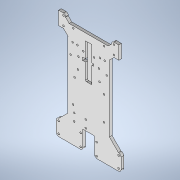
# Autodesk Inventor part: Основа робота
Saved by Autodesk Inventor 2020 (Build 240168000, 168)
## iProperties
Created: 2021-02-28
Part Number: Основа робота
Material: Типовые
Document SubType Name: Обычные детали
Designer: Антон
Density: 1 g/cm^3
Appearance: По умолчанию
Mass: 52.0111 g
Surface Area: 352.197 cm^2
Volume: 52.0111 cm^3
Sheet Metal Rule: По умолчанию
Author: Антон
Autodesk Inventor part; units mm, degrees
ref_plane "YZ Plane" through (0, 0, 0) normal (1, 0, 0) x (0, 1, 0)
ref_plane "XZ Plane" through (0, 0, 0) normal (0, 1, 0) x (-1, 0, 0)
ref_plane "XY Plane" through (0, 0, 0) normal (0, 0, 1) x (1, 0, 0)
sketch "Эскиз1" plane through (0, 0, 0) normal (0, 0, 1) x (1, 0, 0)
  line L0 (0, 0) -> (39, 0)
  line L1 (39, 0) -> (39, 194.6)
  line L2 (39, 194.6) -> (0, 194.6)
  line L3 (0, 194.6) -> (0, 0)
  line L4 (0, 0) -> (-22.05, 0)
  line L5 (-22.05, 0) -> (-22.05, 30.3)
  line L6 (-22.05, 30.3) -> (0, 30.3)
  line L7 (0, 30.3) -> (0, 0)
  line L8 (-22.05, 0) -> (-17.5, 0)
  line L9 (-17.5, 0) -> (-17.5, 4.55)
  line L10 (-17.5, 4.55) -> (-17.5, 25.75)
  circle A0 centre (-17.5, 25.75) radius 1.6
  circle A1 centre (-17.5, 4.55) radius 1.6
  line L11 (39, 0) -> (28, 0)
  line L12 (28, 0) -> (28, 35)
  line L13 (28, 35) -> (39, 35)
  line L14 (39, 35) -> (39, 0)
  line L15 (28, 4) -> (24, 4)
  line L16 (28, 26.9) -> (24, 26.9)
  circle A2 centre (24, 26.9) radius 1.6
  circle A3 centre (24, 4) radius 1.6
  line L17 (39, 154.3) -> (-0.05, 154.3)
  line L18 (-0.05, 154.3) -> (-0.05, 122.8)
  line L19 (-0.05, 122.8) -> (39, 122.8)
  line L20 (39, 122.8) -> (39, 154.3)
  line L21 (-0.05, 154.3) -> (4.95, 154.3)
  line L22 (4.95, 154.3) -> (4.95, 136.3)
  line L23 (4.95, 136.3) -> (-0.05, 136.3)
  line L24 (-0.05, 136.3) -> (-0.05, 154.3)
  line L25 (39, 122.8) -> (18.5177, 122.8)
  line L26 (18.5177, 122.8) -> (18.5177, 132.8)
  line L27 (18.5177, 132.8) -> (39, 132.8)
  line L28 (39, 132.8) -> (39, 122.8)
  line L29 (18.5177, 132.8) -> (9.8575, 127.8)
  line L30 (9.8575, 127.8) -> (4.95, 136.3)
  line L31 (4.95, 136.3) -> (13.6103, 141.3)
  line L32 (13.6103, 141.3) -> (18.5177, 132.8)
  line L33 (18.5177, 122.8) -> (9.8575, 127.8)
  line L34 (13.6103, 141.3) -> (4.95, 154.3)
  line L35 (39, 194.6) -> (39, 154.3)
  circle A4 centre (4.95, 145.3) radius 1.6
  line L36 (18.5177, 132.8) -> (28.7497, 132.8)
  line L37 (28.7497, 132.8) -> (28.7497, 162.65)
  circle A5 centre (28.7497, 162.65) radius 1.6
  line L38 (19.75, 167.25) -> (19.75, 149.25)
  circle A6 centre (19.75, 149.25) radius 1.6
  line L39 (0, 167.25) -> (19.75, 167.25)
  line L40 (19.75, 167.25) -> (17.75, 167.25)
  circle A7 centre (17.75, 167.25) radius 1.6
  line L41 (17.75, 167.25) -> (8.75, 167.25)
  circle A8 centre (8.75, 167.25) radius 1.6
  line L42 (34.9997, 132.8) -> (34.9997, 135.85)
  circle A9 centre (34.9997, 135.85) radius 2.5
  line L43 (39, 137.8498) -> (36.5, 137.8498)
  line L44 (36.5, 137.8498) -> (36.5, 133.8502)
  line L45 (36.5, 133.8502) -> (39, 133.8502)
  line L46 (39, 133.8502) -> (39, 137.8498)
  line L47 (39, 194.6) -> (39, 190.6)
  line L48 (39, 190.6) -> (10, 190.6)
  circle A10 centre (10, 190.6) radius 1.6
  line L49 (39, 194.6) -> (34, 194.6)
  line L50 (34, 194.6) -> (18, 194.6)
  line L51 (0, 181.3) -> (-17.75, 181.3)
  line L52 (-17.75, 181.3) -> (-17.75, 206.3)
  line L53 (-17.75, 206.3) -> (0, 206.3)
  line L54 (0, 206.3) -> (0, 181.3)
  line L55 (-17.75, 193.8) -> (-8.55, 193.8)
  line L56 (-8.55, 202.3) -> (-8.55, 185.3)
  circle A11 centre (-8.55, 202.3) radius 1.6
  circle A12 centre (-8.55, 185.3) radius 1.6
  line L57 (0, 206.3) -> (-4.55, 206.3)
  line L58 (-4.55, 206.3) -> (-4.55, 194.6)
  line L59 (-4.55, 194.6) -> (0, 194.6)
  line L60 (0, 194.6) -> (0, 206.3)
  line L61 (-8.55, 193.8) -> (-8.05, 193.8)
  circle A13 centre (18.5177, 127.8) radius 1.6
  point P0 (0, 30.3)
  point P1 (28, 0)
  point P2 (39, 35)
  point P3 (36.5, 135.85)
  point P4 (36.5, 133.8502)
  point P5 (37.1648, 143.2)
  point P6 (37.75, 137.8498)
  point P7 (36.5, 143.9498)
  point P8 (36.5, 133.8502)
  point P9 (0, 182.1)
  point P10 (0, 181.3)
  point P11 (0, 194.6)
  point P12 (0, 194.6)
  point P13 (-4.55, 206.3)
  dimension "d293" = 5
  dimension "d0" = 39
  dimension "d1" = 194.6
  dimension "d191" = 22.05
  dimension "d192" = 30.3
  dimension "d207" = 4.55
  dimension "d208" = 4.55
  dimension "d209" = 21.2
  dimension "d210" = 11
  dimension "d211" = 35
  dimension "d215" = 4
  dimension "d270" = 39.05
  dimension "d271" = 31.5
  dimension "d273" = 18
  dimension "d274" = 5
  dimension "d276" = 10
  dimension "d277" = 60
  dimension "d278" = 10
  dimension "d280" = 40.3
  dimension "d283" = 10.232
  dimension "d284" = 29.85
  dimension "d285" = 18
  dimension "d286" = 19.75
  dimension "d287" = 27.35
  dimension "d288" = 2
  dimension "d289" = 9
  dimension "d290" = 3.2
  dimension "d292" = 16.482
  dimension "d294" = 3.05
  dimension "d305" = 2.5
  dimension "d309" = 29
  dimension "d310" = 3.2
  dimension "d311" = 3.2
  dimension "d316" = 17.75
  dimension "d317" = 25
  dimension "d320" = 9.2
  dimension "d321" = 3.2
  dimension "d322" = 17
  dimension "d324" = 13.3
  dimension "d325" = 4
  dimension "d333" = 4.55
  dimension "d342" = 0.5
  dimension "d387" = 22.9
  dimension "d388" = 4
  dimension "d404" = 3.2
  constraints: 124 end point, 21 parallel, 15 perpendicular, 14 horizontal, 13 centre point, 13 point on line, 12 coincident, 8 equal radius, 6 midpoint, 3 collinear, 2 vertical, 1 horizontal alignment, 3 other
  measures "d0" distance of L2.end L1.end
  measures "d1" distance of L1.end L0.end
  measures "d191" distance of L5.end L6.end
  measures "d192" distance of L4.end L5.end
  measures "d207" distance of L4.end L8.end
  measures "d208" distance of L8.end L9.end
  measures "d209" distance of L9.end L10.end
  measures "d210" distance of L12.end L13.end
  measures "d211" distance of L11.end L12.end
  measures "d215" distance of L16.start L16.end
  measures "d270" distance of L19.end L18.end
  measures "d271" distance of L18.end L17.end
  measures "d273" distance of L21.end L22.end
  measures "d274" distance between parallel lines of L18 L22
  measures "d276" distance between parallel lines of L25 L27
  measures "d277" angle of L22 L31
  measures "d278" distance between parallel lines of L30 L32
  measures "d280" distance of L1.end L17.start
  measures "d283" distance of L26.end L36.end
  measures "d284" distance of L36.end L37.end
  measures "d285" distance of L38.start L38.end
  measures "d286" distance of L39.start L38.start
  measures "d287" distance between parallel lines of L2 L39
  measures "d288" distance of L38.start L40.end
  measures "d289" distance of L41.start L41.end
  measures "d290" diameter of A2
  measures "d292" distance between parallel lines of L26 L42
  measures "d294" distance of L42.start L42.end
  measures "d305" distance of L45.end L44.end
  measures "d309" distance of L47.end L48.end
  measures "d310" diameter of A8
  measures "d311" diameter of A10
  measures "d316" distance of L52.end L53.end
  measures "d317" distance of L51.end L52.end
  measures "d320" distance of L55.end L55.start
  measures "d321" diameter of A11
  measures "d322" distance of L56.end L56.start
  measures "d324" distance between parallel lines of L2 L51
  measures "d325" distance from line of L49.end L48
  measures "d333" distance of L59.end L58.end
  measures "d342" distance of L61.end L55.end
  measures "d387" distance of A3.centre A2.centre
  measures "d388" distance between parallel lines of L0 L15
  measures "d404" diameter of A4
extrude "Выдавливание1" add sketch "Эскиз1" along normal blind 5 contours L3 L19 L1 L13 L12 L0 | L4 L5 L6 L3 | L3 L23 L30 L33 L19 | L3 L17 L22 A4 L23 | L26 A13 L27 L1 L19 | L33 L29 L26 A13 | L3 L39 A8 A7 L38 L17 | L31 L32 L29 L30 | L22 A4 L34 L31 | L27 L42 A9 L45 L1 | L3 L2 L1 L17 L38 L39 A7 A8 | L17 L37 L27 L32 L34 | L45 A9 L43 L1 | L27 L37 L17 L1 L43 A9 L42 | L51 L52 L53 L58 L59 L3 | L44 A9 | A9 L44
mirror "Зеркальное отражение1" about plane through (39, 35, 0) normal (1, 0, 0) of "Выдавливание1"
sketch "Эскиз18" plane through (0, 0, 5) normal (0, 0, 1) x (1, 0, 0)
  line L0 (39, 194.6) -> (39, 111.75)
  line L1 (39, 111.75) -> (67.8, 111.75)
  line L2 (39, 111.75) -> (12.6, 111.75)
  line L3 (39, 111.75) -> (39, 66.05)
  line L4 (39, 66.05) -> (67.8, 66.05)
  line L5 (39, 66.05) -> (9.6, 66.05)
  line L6 (-4.55, 194.6) -> (82.55, 194.6) projected
  dimension "d218" = 82.85
  dimension "d219" = 28.8
  dimension "d220" = 26.4
  dimension "d221" = 45.7
  dimension "d222" = 28.8
  dimension "d223" = 29.4
  constraints: 12 end point, 4 horizontal, 2 vertical, 1 midpoint
  measures "d218" distance of L0.start L0.end
  measures "d219" distance of L0.end L1.end
  measures "d220" distance of L0.end L2.end
  measures "d221" distance of L0.end L3.end
  measures "d222" distance of L3.end L4.end
  measures "d223" distance of L3.end L5.end
hole "Отверстие10" at (67.8, 111.75, 5) at (12.6, 111.75, 5) at (9.6, 66.05, 5) at (67.8, 66.05, 5) direction (0, 0, -1) diameter 3.2 end through all
fillet "Сопряжение2" radius 5.05 6 edges at (-22.05, 30.3, 2.5) (-22.05, 0, 2.5) (28, 0, 2.5) (50, 0, 2.5) (100.05, 0, 2.5) (100.05, 30.3, 2.5)
sketch "Эскиз19" plane through (0, 0, 0) normal (0, 0, -1) x (-1, 0, 0)
  circle A0 centre (-86.55, 202.3) radius 1.6 projected
  circle A1 centre (-86.55, 202.3) radius 1.6 projected
  line L0 (-85.0489, 204.9) -> (-83.5478, 202.3)
  line L1 (-83.5478, 202.3) -> (-85.0489, 199.7)
  line L2 (-85.0489, 199.7) -> (-88.0511, 199.7)
  line L3 (-88.0511, 199.7) -> (-89.5522, 202.3)
  line L4 (-89.5522, 202.3) -> (-88.0511, 204.9)
  line L5 (-88.0511, 204.9) -> (-85.0489, 204.9)
  line L6 (-82.55, 206.3) -> (-95.75, 206.3) projected
  dimension "d365" = 5.2
  constraints: 12 end point, 1 coincident, 1 parallel, 13 other
  measures "d365" distance between parallel lines of L2 L5
extrude "Выдавливание7" cut sketch "Эскиз19" against normal blind 2.6 contours A0 | L0 L1 L2 L3 L4 L5
chamfer "Фаска1" distance 17 angle 45 2 edges at (0, 30.3, 2.5) (78, 30.3, 2.5)
sketch "Эскиз21" plane through (0, 0, 5) normal (0, 0, 1) x (1, 0, 0)
  line L0 (39, 194.6) -> (39, 178.615)
  line L1 (45.05, 178.615) -> (32.95, 178.615)
  line L2 (32.95, 178.615) -> (32.95, 115.75)
  line L3 (32.95, 115.75) -> (45.05, 115.75)
  line L4 (45.05, 115.75) -> (45.05, 178.615)
  line L5 (43, 117.8) -> (35, 117.8) construction
  line L6 (43, 115.75) -> (35, 115.75)
  line L7 (35, 119.85) -> (43, 119.85)
  arc A0 (43, 115.75) -> (43, 119.85) centre (43, 117.8) ccw
  arc A1 (35, 119.85) -> (35, 115.75) centre (35, 117.8) ccw
  line L8 (-4.55, 194.6) -> (82.55, 194.6) projected
  point P0 (0, 0)
  point P1 (39, 117.8)
  point P2 (32.95, 117.8)
  point P3 (35, 115.75)
  point P4 (43, 115.75)
  point P5 (45.05, 117.8)
  dimension "d297" = 12.1
  dimension "d298" = 62.865
  dimension "d299" = 15.985
  dimension "d307" = 4.1
  constraints: 18 end point, 6 tangent, 4 point on circle, 3 midpoint, 3 parallel, 2 centre point, 2 perpendicular, 1 collinear, 1 horizontal, 1 vertical
  measures "d297" distance of L3.end L2.end
  measures "d298" distance of L2.end L1.end
  measures "d299" distance of L0.start L0.end
  measures "d307" distance between parallel lines of L3 L7
extrude "Выдавливание9" cut sketch "Эскиз21" against normal blind 4 contours L4 A0 L7 A1 L2 L1 | A0 L3 A1 L7
chamfer "Фаска2" distance 3 angle 45 1 edges at (39, 178.615, 5)
chamfer "Фаска3" distance 8.55 angle 45 2 edges at (0, 181.3, 2.5) (78, 181.3, 2.5)
fillet "Сопряжение8" radius 4 2 edges at (-4.55, 206.3, 2.5) (82.55, 206.3, 2.5)
chamfer "Фаска5" distance 6.8 angle 45 2 edges at (-4.55, 194.6, 2.5) (82.55, 194.6, 2.5)
sketch "Эскиз28" plane through (0, 0, 5) normal (0, 0, 1) x (1, 0, 0)
  line L0 (50, 5.05) -> (50, 35) projected
  line L1 (28, 35) -> (50, 35) projected
  line L2 (33.55, 39.504) -> (11.8, 39.504)
  line L3 (11.8, 39.504) -> (11.8, 53.512)
  line L4 (11.8, 53.512) -> (33.55, 53.512)
  line L5 (33.55, 53.512) -> (33.55, 39.504)
  point P0 (0, 0)
  dimension "d400" = 21.75
  dimension "d401" = 14.008
  dimension "d402" = 4.504
  dimension "d403" = 16.45
  constraints: 8 end point, 2 parallel, 1 horizontal, 1 perpendicular
  measures "d400" distance of L3.end L4.end
  measures "d401" distance of L2.end L3.end
  measures "d402" distance between parallel lines of L1 L2
  measures "d403" distance between parallel lines of L0 L5
hole "Отверстие12" at (33.55, 39.504, 5) at (11.8, 39.504, 5) at (33.55, 53.512, 5) at (11.8, 53.512, 5) direction (0, 0, -1) diameter 3.2 end through all
pattern_sketch "Массив по эскизу1" of "Выдавливание7" from (86.55, 202.3, 0) copies at (24, 26.9, 0) at (24, 4, 0) at (-17.5, 25.75, 0) at (-17.5, 4.55, 0) at (54, 26.9, 0) at (54, 4, 0) at (95.5, 4.55, 0) at (95.5, 25.75, 0) at (67.8, 66.05, 0) at (9.6, 66.05, 0) at (67.8, 111.75, 0) at (12.6, 111.75, 0) at (19.75, 149.25, 0) at (4.95, 145.3, 0) at (58.25, 149.25, 0) at (73.05, 145.3, 0) at (69.25, 167.25, 0) at (60.25, 167.25, 0) at (49.2503, 162.65, 0) at (28.7497, 162.65, 0) at (17.75, 167.25, 0) at (8.75, 167.25, 0) at (10, 190.6, 0) at (-8.55, 185.3, 0) at (-8.55, 202.3, 0) at (86.55, 185.3, 0) at (68, 190.6, 0) at (33.55, 53.512, 0) at (33.55, 39.504, 0) at (11.8, 39.504, 0) at (11.8, 53.512, 0) at (18.5177, 127.8, 0) at (59.4823, 127.8, 0)
sketch "Эскиз29" plane through (0, 0, 5) normal (0, 0, 1) x (1, 0, 0)
  line L0 (48.05, 147.7075) -> (45.05, 147.7075)
  line L1 (45.05, 147.7075) -> (45.05, 151.7075)
  line L2 (45.05, 151.7075) -> (48.05, 151.7075)
  line L3 (48.05, 151.7075) -> (48.05, 147.7075)
  line L4 (45.05, 181.615) -> (45.05, 117.8) projected
  line L5 (32.95, 146.9575) -> (27.45, 146.9575)
  line L6 (27.45, 146.9575) -> (27.45, 152.4575)
  line L7 (27.45, 152.4575) -> (32.95, 152.4575)
  line L8 (32.95, 152.4575) -> (32.95, 146.9575)
  line L9 (32.95, 117.8) -> (32.95, 181.615) projected
  point P0 (0, 0)
  point P1 (45.05, 149.7075)
  point P2 (32.95, 149.7075)
  dimension "d405" = 3
  dimension "d406" = 4
  dimension "d407" = 5.5
  dimension "d408" = 5.5
  constraints: 16 end point, 4 midpoint, 4 parallel, 2 horizontal, 2 perpendicular
  measures "d405" distance of L1.end L2.end
  measures "d406" distance of L0.end L1.end
  measures "d407" distance of L5.start L5.end
  measures "d408" distance of L5.end L6.end
extrude "Выдавливание13" cut sketch "Эскиз29" against normal through all
sketch "Эскиз25" plane through (0, 0, 0) normal (0, 0, -1) x (-1, 0, 0)
  circle A0 centre (-24, 26.9) radius 1.6 projected
  circle A1 centre (-24, 4) radius 1.6 projected
  circle A2 centre (17.5, 25.75) radius 1.6 projected
  circle A3 centre (17.5, 4.55) radius 1.6 projected
  circle A4 centre (-54, 26.9) radius 1.6 projected
  circle A5 centre (-54, 4) radius 1.6 projected
  circle A6 centre (-95.5, 4.55) radius 1.6 projected
  circle A7 centre (-95.5, 25.75) radius 1.6 projected
  circle A8 centre (-67.8, 66.05) radius 1.6 projected
  circle A9 centre (-9.6, 66.05) radius 1.6 projected
  circle A10 centre (-67.8, 111.75) radius 1.6 projected
  circle A11 centre (-12.6, 111.75) radius 1.6 projected
  circle A12 centre (-19.75, 149.25) radius 1.6 projected
  circle A13 centre (-4.95, 145.3) radius 1.6 projected
  circle A14 centre (-58.25, 149.25) radius 1.6 projected
  circle A15 centre (-73.05, 145.3) radius 1.6 projected
  circle A16 centre (-69.25, 167.25) radius 1.6 projected
  circle A17 centre (-60.25, 167.25) radius 1.6 projected
  circle A18 centre (-49.2503, 162.65) radius 1.6 projected
  circle A19 centre (-28.7497, 162.65) radius 1.6 projected
  circle A20 centre (-17.75, 167.25) radius 1.6 projected
  circle A21 centre (-8.75, 167.25) radius 1.6 projected
  circle A22 centre (-10, 190.6) radius 1.6 projected
  circle A23 centre (8.55, 185.3) radius 1.6 projected
  circle A24 centre (8.55, 202.3) radius 1.6 projected
  circle A25 centre (-86.55, 185.3) radius 1.6 projected
  circle A26 centre (-68, 190.6) radius 1.6 projected
  circle A27 centre (-33.55, 53.512) radius 1.6 projected
  circle A28 centre (-33.55, 39.504) radius 1.6 projected
  circle A29 centre (-11.8, 39.504) radius 1.6 projected
  circle A30 centre (-11.8, 53.512) radius 1.6 projected
  circle A31 centre (-18.5177, 127.8) radius 1.6 projected
  circle A32 centre (-59.4823, 127.8) radius 1.6 projected
  circle A33 centre (-18.5177, 127.8) radius 1.6 projected
  point P0 (0, 0)
  point P1 (-54, 4)
  point P2 (-95.5, 4.55)
  point P3 (-95.5, 25.75)
  constraints: 33 coincident
equation "\"Радиус_гибки\" = Толщина"
equation "\"Ширина_просечки\" = Толщина"
equation "\"Глубина_просечки\" = 0.5 * Толщина"
equation "\"Размер_просечки\" = 4 * Толщина"
equation "\"Мин_остаток\" = 2 * Толщина"
equation "\"Радиус_перехода\" = Радиус_гибки"
equation "\"Радиус_Якоби\" = Толщина"
equation "\"Размер_зазора\" = Толщина"
equation "\"Гайка_М3_з\" = 5.6"
equation "\"d130\" = 5.6"
equation "\"Толщина\" = 0.5"
